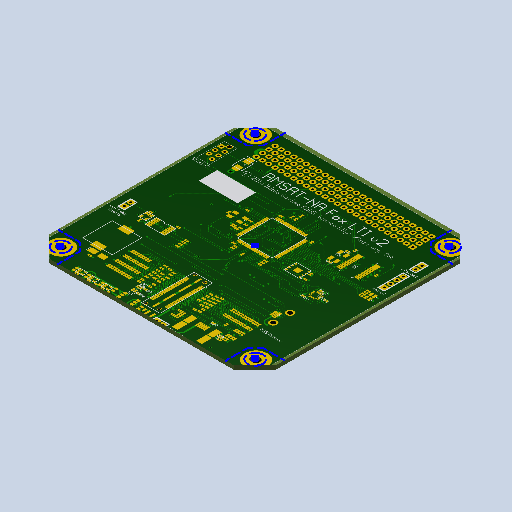
# Autodesk Inventor part: PCB_LIHU
Saved by Autodesk Inventor 2023 (Build 270158000, 158)
## iProperties
Created: 2011-02-14
Part Number: PCB_LIHU
Material: FR4
Document SubType Name: Modeling
Designer: Robert Davis
Mass: 35.4838 g
Surface Area: 181.406 cm^2
Volume: 13.888 cm^3
Density: 2.555 g/cm^3
Appearance: Olive Green
Author: Robert Davis
Autodesk Inventor part; units mm, degrees
ref_plane "XY Plane" through (0, 0, 0) normal (0, 0, 1) x (1, 0, 0)
sketch "Sketch1" plane through (0, 0, 0) normal (0, 0, 1) x (1, 0, 0)
  line L0 (-46, 46) -> (46, 46)
  line L1 (46, 46) -> (46, -46)
  line L2 (46, -46) -> (-46, -46)
  line L3 (-46, -46) -> (-46, 46)
  circle A0 centre (39.5, 39.5) radius 1.5875
  circle A1 centre (-39.5, 39.5) radius 1.5875
  circle A2 centre (-39.5, -39.5) radius 1.5875
  circle A3 centre (39.5, -39.5) radius 1.5875
  line L4 (0, 10.5587) -> (0, 0)
  line L5 (0, 0) -> (12.3531, 0)
  circle A4 centre (-39.5, 39.5) radius 3.175 construction
  line L6 (-38, 44.6281) -> (-38, 37.8613) construction
  dimension "d0" = 92
  dimension "d1" = 92
  dimension "d508" = 3.175
  dimension "d509" = 79
  dimension "d510" = 79
  dimension "d511" = 6.35
  dimension "d515" = 76
  constraints: 14 end point, 5 centre point, 4 vertical, 3 equal radius, 3 horizontal, 2 coincident, 2 horizontal alignment, 2 symmetric about line, 2 vertical alignment, 2 other
  measures "d0" distance of L0.start L0.end
  measures "d1" distance of L0.end L1.end
  measures "d508" diameter of A1
  measures "d509" distance of A0.centre A1.centre
  measures "d510" distance of A3.centre A0.centre
  measures "d511" diameter of A4
  measures "d515" diameter of L6 L4
extrude "Extrusion1" add sketch "Sketch1" along normal blind 1.5875
ref_plane "Work Plane_ConnX" through (-32, 0, 0) normal (1, 0, 0) x (0, 1, 0)
ref_plane "Work Plane_ConnY" through (0, 0, 0) normal (0, 1, 0) x (-1, 0, 0)
sketch "Sketch9" plane through (0, 0, 1.5875) normal (0, 0, 1) x (1, 0, 0)
  line L0 (46, 46) -> (46, -46) projected
  line L1 (58.5598, -32) -> (-58.5598, -32)
  circle A0 centre (-2.667, -21.935) radius 0.51
  circle A1 centre (-2.667, -42.065) radius 0.51
  line L2 (0, 26.5598) -> (0, -90.5598) construction
  point P0 (0, 0)
  point P1 (0, -32)
  dimension "d134" = 20.13
  dimension "d136" = 2.667
  dimension "d138" = 1.02
  dimension "d141" = 180
  dimension "d350" = 32
  dimension "d351" = 0
  constraints: 4 end point, 2 centre point, 2 midpoint, 2 perpendicular, 1 symmetric about line, 1 other
  measures "d134" distance of A0.centre A1.centre
  measures "d136" distance from line of L2 A0.centre
  measures "d138" diameter of A0
  measures "d141" angle of L0 L2
  measures "d350" distance of point (0, 0) point (0, -32)
  measures "d351" horizontal distance of point (0, 0) point (0, -32)
extrude "Holes_Conn_Zminus" cut sketch "Sketch9" against normal through all
sketch "Sketch22" plane through (0, 0, 1.5875) normal (0, 0, 1) x (1, 0, 0)
  line L0 (46, 46) -> (46, -46) projected
  line L1 (0, -1.0026) -> (0, -62.9974) construction
  line L2 (62.8115, -32) -> (-62.8115, -32)
  circle A0 centre (2.032, -22.7608) radius 0.51
  circle A1 centre (2.032, -41.2392) radius 0.51
  point P0 (46, -35)
  point P1 (46, 35)
  point P2 (0, 0)
  point P3 (0, -32)
  dimension "d282" = 180
  dimension "d283" = 18.4785
  dimension "d284" = 1.02
  dimension "d285" = 2.032
  dimension "d352" = 32
  dimension "d353" = 0
  constraints: 4 end point, 2 centre point, 2 midpoint, 1 perpendicular, 1 other
  measures "d282" angle of L0 L1
  measures "d283" distance of A0.centre A1.centre
  measures "d284" diameter of A1
  measures "d285" distance from line of L1 A0.centre
  measures "d352" distance of point (0, 0) point (0, -32)
  measures "d353" horizontal distance of point (0, 0) point (0, -32)
extrude "Holes_Conn_Zplus" cut sketch "Sketch22" against normal through all
chamfer "Chamfer4" distance 8.5 angle 45 4 edges at (-46, 46, 0.7937) (46, 46, 0.7937) (46, -46, 0.7937) (-46, -46, 0.7937)
sketch "Sketch31" plane through (0, 0, 1.5875) normal (0, 0, 1) x (1, 0, 0)
  circle A0 centre (39.5, -39.5) radius 3.175
  circle A1 centre (39.5, 39.5) radius 3.175
  circle A2 centre (-39.5, 39.5) radius 3.175
  circle A3 centre (-39.5, -39.5) radius 3.175
  point P0 (0, 0)
  dimension "d5" = 0
  dimension "d516" = 6.35
  constraints: 4 centre point, 3 equal radius
  measures "d516" diameter of A1
sketch "Sketch32" plane through (0, 0, 1.5875) normal (0, 0, 1) x (1, 0, 0)
  line L0 (34, -46) -> (34, -37.2218)
  line L1 (34, -37.2218) -> (37.2218, -34)
  line L2 (37.2218, -34) -> (46, -34)
  line L3 (46, 34) -> (37.2218, 34)
  line L4 (37.2218, 34) -> (34, 37.2218)
  line L5 (34, 37.2218) -> (34, 46)
  line L6 (-34, 46) -> (-34, 37.2218)
  line L7 (-34, 37.2218) -> (-37.2218, 34)
  line L8 (-37.2218, 34) -> (-46, 34)
  line L9 (-34, -46) -> (-34, -37.2218)
  line L10 (-34, -37.2218) -> (-37.2218, -34)
  line L11 (-37.2218, -34) -> (-46, -34)
  point P0 (39.5, -39.5)
  point P1 (0, 0)
  dimension "d5" = 0
  dimension "d519" = 5.5
  dimension "d520" = 5.5
  constraints: 24 end point, 10 equal length, 4 perpendicular, 2 parallel
  measures "d519" distance from line of point (39.5, -39.5) L0
  measures "d520" distance from line of point (39.5, -39.5) L1
sketch "Sketch33" plane through (0, 0, 1.5875) normal (0, 0, 1) x (1, 0, 0)
  line L0 (37.5, -46) -> (-37.5, -46) projected
  line L1 (46, 37.5) -> (46, -37.5) projected
  line L2 (-37.5, 46) -> (37.5, 46) projected
  line L3 (-45.0742, 44.5) -> (45.0742, 44.4997) construction
  line L4 (45.0742, 44.4997) -> (45.074, -47.5003) construction
  line L5 (45.074, -47.5003) -> (-45.0745, -47.5) construction
  line L6 (-45.0745, -47.5) -> (-45.0742, 44.5) construction
  point P0 (0, 0)
  point P1 (45.0741, -1.5003)
  point P2 (46, 0)
  point P3 (0, 46)
  point P4 (0, 44.4999)
  dimension "d537" = 92
  dimension "d557" = 1.5
  constraints: 4 midpoint, 1 vertical alignment, 2 other
  measures "d537" distance of L4.end L3.end
  measures "d557" distance from line of L0 L5.end
decal "Decal4"
sketch "Sketch34" plane through (0, 0, 0) normal (0, 0, -1) x (-1, 0, 0)
  line L0 (37.5, 46) -> (-37.5, 46) projected
  line L1 (-37.5, -46) -> (37.5, -46) projected
  line L2 (-44.9565, 44.5) -> (44.9565, 44.5) construction
  line L3 (44.9565, 44.5) -> (44.9565, -47.5) construction
  line L4 (44.9565, -47.5) -> (-44.9565, -47.5) construction
  line L5 (-44.9565, -47.5) -> (-44.9565, 44.5) construction
  point P0 (0, 0)
  point P1 (0, 44.5)
  point P2 (0, 46)
  dimension "d559" = 92
  dimension "d564" = 1.5
  constraints: 2 midpoint, 1 horizontal alignment, 1 vertical alignment, 2 other
  measures "d559" distance of L2.end L3.end
  measures "d564" distance from line of L1 L4.end
decal "Decal5"
body "Solid1"
